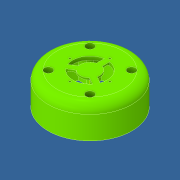
# Autodesk Inventor part: MotorCoverN24_3
Saved by Autodesk Inventor 2016 (Build 200138000, 138)
## iProperties
Created: 2015-09-10
Part Number: MotorCoverN24_3
Material: ABS-Kunststoff
Document SubType Name: Modeling
Designer: 4ndreas
Density: 1.06 g/cm^3
Appearance: Glatt - grün
Mass: 119.697 g
Surface Area: 331.914 cm^2
Volume: 112.922 cm^3
Author: 4ndreas
Autodesk Inventor part; units mm, degrees
ref_plane "YZ Plane" through (0, 0, 0) normal (1, 0, 0) x (0, 1, 0)
ref_plane "XZ Plane" through (0, 0, 0) normal (0, 1, 0) x (-1, 0, 0)
sketch "Skizze1" plane through (0, 0, 0) normal (0, 0, 1) x (1, 0, 0)
  line L0 (24.616, 19.6663) -> (20.7123, 20.7123) projected
  line L1 (20.7123, 20.7123) -> (19.6663, 24.616) projected
  line L2 (19.6663, 24.616) -> (22.524, 27.4737) projected
  line L3 (22.524, 27.4737) -> (26.4277, 26.4277) projected
  line L4 (26.4277, 26.4277) -> (27.4737, 22.524) projected
  line L5 (27.4737, 22.524) -> (24.616, 19.6663) projected
  line L6 (-24.616, -19.6663) -> (-20.7123, -20.7123) projected
  line L7 (-20.7123, -20.7123) -> (-19.6663, -24.616) projected
  line L8 (-19.6663, -24.616) -> (-22.524, -27.4737) projected
  line L9 (-22.524, -27.4737) -> (-26.4277, -26.4277) projected
  line L10 (-26.4277, -26.4277) -> (-27.4737, -22.524) projected
  line L11 (-27.4737, -22.524) -> (-24.616, -19.6663) projected
  line L12 (-20.7123, 20.7123) -> (-24.616, 19.6663) projected
  line L13 (-24.616, 19.6663) -> (-27.4737, 22.524) projected
  line L14 (-27.4737, 22.524) -> (-26.4277, 26.4277) projected
  line L15 (-26.4277, 26.4277) -> (-22.524, 27.4737) projected
  line L16 (-22.524, 27.4737) -> (-19.6663, 24.616) projected
  line L17 (-19.6663, 24.616) -> (-20.7123, 20.7123) projected
  line L18 (19.6663, -24.616) -> (20.7123, -20.7123) projected
  line L19 (20.7123, -20.7123) -> (24.616, -19.6663) projected
  line L20 (24.616, -19.6663) -> (27.4737, -22.524) projected
  line L21 (27.4737, -22.524) -> (26.4277, -26.4277) projected
  line L22 (26.4277, -26.4277) -> (22.524, -27.4737) projected
  line L23 (22.524, -27.4737) -> (19.6663, -24.616) projected
  arc A0 (-23.57, 19.32) -> (-19.32, 23.57) centre (-23.57, 23.57) ccw projected
  line L24 (-19.32, 23.57) -> (-19.32, 32.18) projected
  line L25 (-19.32, 32.18) -> (19.32, 32.18) projected
  line L26 (19.32, 32.18) -> (19.32, 23.57) projected
  arc A1 (19.32, 23.57) -> (23.57, 19.32) centre (23.57, 23.57) ccw projected
  line L27 (23.57, 19.32) -> (32.18, 19.32) projected
  line L28 (32.18, 19.32) -> (32.18, -19.32) projected
  line L29 (32.18, -19.32) -> (23.57, -19.32) projected
  arc A2 (23.57, -19.32) -> (19.32, -23.57) centre (23.57, -23.57) ccw projected
  line L30 (19.32, -23.57) -> (19.32, -32.18) projected
  line L31 (19.32, -32.18) -> (-19.32, -32.18) projected
  line L32 (-19.32, -32.18) -> (-19.32, -23.57) projected
  arc A3 (-19.32, -23.57) -> (-23.57, -19.32) centre (-23.57, -23.57) ccw projected
  line L33 (-23.57, -19.32) -> (-32.18, -19.32) projected
  line L34 (-32.18, -19.32) -> (-32.18, 19.32) projected
  line L35 (-32.18, 19.32) -> (-23.57, 19.32) projected
  circle A4 centre (0, 0) radius 47.5
  circle A5 centre (23.57, -23.57) radius 2
  circle A6 centre (23.57, 23.57) radius 2
  circle A7 centre (-23.57, 23.57) radius 2
  circle A8 centre (-23.57, -23.57) radius 2
  arc A9 (32.18, -19.32) -> (32.18, 19.32) centre (0, 0) ccw
  arc A10 (-19.32, -32.18) -> (19.32, -32.18) centre (0, 0) ccw
  arc A11 (-32.18, 19.32) -> (-32.18, -19.32) centre (0, 0) ccw
  arc A12 (19.32, 32.18) -> (-19.32, 32.18) centre (0, 0) ccw
  point P0 (0, 0)
  dimension "d0" = 4
  dimension "d40" = 95
  constraints: 9 centre point, 8 coincident, 8 point on circle, 3 equal radius
  measures "d0" diameter of A5
  measures "d40" diameter of A4
extrude "Extrusion1" add sketch "Skizze1" along normal blind 32 contours L0 L1 L2 L3 L4 L5 | L6 L7 L8 L9 L10 L11 | L12 L13 L14 L15 L16 L17 | L18 L19 L20 L21 L22 L23 | A4
ref_plane "Arbeitsebene1" through (0, 0, 0) normal (1, 0, 0) x (0, 0, 1)
sketch "Skizze9" plane through (0, 0, 32) normal (0, 0, 1) x (1, 0, 0)
  circle A0 centre (23.57, -23.57) radius 2 projected
  circle A1 centre (-23.57, 23.57) radius 2 projected
  circle A2 centre (-23.57, -23.57) radius 2 projected
  circle A3 centre (23.57, 23.57) radius 2 projected
  circle A4 centre (0, 0) radius 47.5 projected
  line L0 (32.18, -19.32) -> (23.57, -19.32) projected
  arc A5 (23.57, -19.32) -> (19.32, -23.57) centre (23.57, -23.57) ccw projected
  line L1 (19.32, -23.57) -> (19.32, -32.18) projected
  arc A6 (-19.32, -32.18) -> (19.32, -32.18) centre (0, 0) ccw projected
  line L2 (-19.32, -32.18) -> (-19.32, -23.57) projected
  arc A7 (-19.32, -23.57) -> (-23.57, -19.32) centre (-23.57, -23.57) ccw projected
  line L3 (-23.57, -19.32) -> (-32.18, -19.32) projected
  arc A8 (-32.18, 19.32) -> (-32.18, -19.32) centre (0, 0) ccw projected
  line L4 (-32.18, 19.32) -> (-23.57, 19.32) projected
  arc A9 (-23.57, 19.32) -> (-19.32, 23.57) centre (-23.57, 23.57) ccw projected
  line L5 (-19.32, 23.57) -> (-19.32, 32.18) projected
  arc A10 (19.32, 32.18) -> (-19.32, 32.18) centre (0, 0) ccw projected
  line L6 (19.32, 32.18) -> (19.32, 23.57) projected
  arc A11 (19.32, 23.57) -> (23.57, 19.32) centre (23.57, 23.57) ccw projected
  line L7 (23.57, 19.32) -> (32.18, 19.32) projected
  arc A12 (32.18, -19.32) -> (32.18, 19.32) centre (0, 0) ccw projected
  point P0 (0, 0)
extrude "Extrusion6" add sketch "Skizze9" along normal blind 4 contours A4 | L0 A5 L1 A6 L2 A7 L3 A8 L4 A9 L5 A10 L6 A11 L7 A12
fillet "Rundung3" radius 10 1 edges at (-47.5, 0, 36)
sketch "Skizze10" plane through (0, 0, 0) normal (0, 0, -1) x (-1, 0, 0)
  circle A0 centre (-23.57, -23.57) radius 2 projected
  circle A1 centre (23.57, 23.57) radius 2 projected
  circle A2 centre (23.57, -23.57) radius 2 projected
  circle A3 centre (-23.57, 23.57) radius 2 projected
  line L0 (-23.57, -19.32) -> (-32.18, -19.32) projected
  arc A4 (-32.18, 19.32) -> (-32.18, -19.32) centre (0, 0) ccw projected
  line L1 (-32.18, 19.32) -> (-23.57, 19.32) projected
  arc A5 (-23.57, 19.32) -> (-19.32, 23.57) centre (-23.57, 23.57) ccw projected
  line L2 (-19.32, 23.57) -> (-19.32, 32.18) projected
  arc A6 (19.32, 32.18) -> (-19.32, 32.18) centre (0, 0) ccw projected
  line L3 (19.32, 32.18) -> (19.32, 23.57) projected
  arc A7 (19.32, 23.57) -> (23.57, 19.32) centre (23.57, 23.57) ccw projected
  line L4 (23.57, 19.32) -> (32.18, 19.32) projected
  arc A8 (32.18, -19.32) -> (32.18, 19.32) centre (0, 0) ccw projected
  line L5 (32.18, -19.32) -> (23.57, -19.32) projected
  arc A9 (23.57, -19.32) -> (19.32, -23.57) centre (23.57, -23.57) ccw projected
  line L6 (19.32, -23.57) -> (19.32, -32.18) projected
  arc A10 (-19.32, -32.18) -> (19.32, -32.18) centre (0, 0) ccw projected
  line L7 (-19.32, -32.18) -> (-19.32, -23.57) projected
  arc A11 (-19.32, -23.57) -> (-23.57, -19.32) centre (-23.57, -23.57) ccw projected
  circle A12 centre (0, 0) radius 47.5 projected
  point P0 (0, 0)
fillet "Rundung4" radius 5 12 edges at (20.5648, 20.5648, 32) (27.875, 19.32, 32) (19.32, 27.875, 32) (19.32, -27.875, 32) (27.875, -19.32, 32) (20.5648, -20.5648, 32) (-27.875, -19.32, 32) (-19.32, -27.875, 32) (-20.5648, -20.5648, 32) (-19.32, 27.875, 32) (-27.875, 19.32, 32) (-20.5648, 20.5648, 32)
sketch "Skizze11" plane through (0, 0, 36) normal (0, 0, 1) x (1, 0, 0)
  circle A0 centre (23.57, -23.57) radius 2 projected
  circle A1 centre (-23.57, 23.57) radius 2 projected
  circle A2 centre (-23.57, -23.57) radius 2 projected
  circle A3 centre (23.57, 23.57) radius 2 projected
  circle A4 centre (0, 0) radius 37.5 projected
  point P0 (0, 0)
hole "Bohrung2" at (-23.57, 23.57, 36) at (23.57, 23.57, 36) at (23.57, -23.57, 36) at (-23.57, -23.57, 36) direction (0, 0, -1) diameter 4.2 end through all counterbore diameter 9 counterbore depth 6
sketch "Skizze12" plane through (0, 0, 36) normal (0, 0, 1) x (1, 0, 0)
  line L0 (0, -28.2843) -> (28.2843, 0)
  line L1 (28.2843, 0) -> (0, 28.2843)
  line L2 (0, 28.2843) -> (-28.2843, 0)
  line L3 (-28.2843, 0) -> (0, -28.2843)
  line L4 (0, -28.2843) -> (0, 28.2843) construction
  line L5 (28.2843, 0) -> (-28.2843, 0) construction
  arc A0 (25.2121, 27.7597) -> (-25.2121, 27.7597) centre (0, 0) ccw projected
  circle A1 centre (23.57, 23.57) radius 2.1 projected
  circle A2 centre (-23.57, 23.57) radius 2.1 projected
  line L6 (0, -22.6274) -> (22.6274, 0) construction
  line L7 (22.6274, 0) -> (0, 22.6274) construction
  line L8 (0, 22.6274) -> (-22.6274, 0) construction
  line L9 (-22.6274, 0) -> (0, -22.6274) construction
  line L10 (0, -22.6274) -> (0, 22.6274) construction
  line L11 (22.6274, 0) -> (-22.6274, 0) construction
  circle A3 centre (0, 22.6274) radius 1.25
  circle A4 centre (22.6274, 0) radius 1.25
  circle A5 centre (0, -22.6274) radius 1.25
  circle A6 centre (-22.6274, 0) radius 1.25
  circle A7 centre (0, 0) radius 19.5
  circle A8 centre (0, 0) radius 11
  line L12 (-3.1274, 10.5461) -> (3.1274, 10.5461)
  line L13 (3.1274, 10.5461) -> (3.1274, 19.5)
  line L14 (3.1274, 19.5) -> (-3.1274, 19.5)
  line L15 (-3.1274, 19.5) -> (-3.1274, 10.5461)
  line L16 (-3.1274, 10.5461) -> (3.1274, 19.5) construction
  line L17 (3.1274, 10.5461) -> (-3.1274, 19.5) construction
  line L18 (0, 0) -> (-16.8875, -9.75) construction
  line L19 (-15.3238, -12.4584) -> (-7.5694, -7.9814)
  line L20 (-7.5694, -7.9814) -> (-10.6969, -2.5646)
  line L21 (-10.6969, -2.5646) -> (-18.4512, -7.0416)
  line L22 (-18.4512, -7.0416) -> (-15.3238, -12.4584)
  line L23 (-15.3238, -12.4584) -> (-10.6969, -2.5646) construction
  line L24 (-7.5694, -7.9814) -> (-18.4512, -7.0416) construction
  line L25 (0, 0) -> (16.8875, -9.75) construction
  line L26 (15.3238, -12.4584) -> (7.5694, -7.9814)
  line L27 (7.5694, -7.9814) -> (10.6969, -2.5646)
  line L28 (10.6969, -2.5646) -> (18.4512, -7.0416)
  line L29 (18.4512, -7.0416) -> (15.3238, -12.4584)
  line L30 (15.3238, -12.4584) -> (10.6969, -2.5646) construction
  line L31 (7.5694, -7.9814) -> (18.4512, -7.0416) construction
  point P0 (0, 0)
  point P1 (0, 15.023)
  point P2 (-13.0103, -7.5115)
  point P3 (13.0103, -7.5115)
  dimension "d52" = 40
  dimension "d53" = 32
  dimension "d54" = 2.5
  dimension "d55" = 0.5
  dimension "d56" = 22
  dimension "d57" = 120
  dimension "d58" = 120
  constraints: 64 end point, 12 midpoint, 10 parallel, 7 point on circle, 6 centre point, 6 coincident, 5 perpendicular, 4 equal length, 4 point on line, 3 equal radius, 2 collinear, 2 horizontal, 1 tangent, 1 vertical
  measures "d52" distance between parallel lines of L3 L1
  measures "d53" distance between parallel lines of L9 L7
  measures "d54" diameter of A3
  measures "d55" distance edge to line of A7 L1
  measures "d56" diameter of A8
  measures "d57" angle of L18 L4
  measures "d58" angle of L25 L18
extrude "Extrusion7" cut sketch "Skizze12" against normal through all contours A3 | A4 | A5 | A6 | A7 L28 A8 L13 | L13 A8 L15 A7 | A7 L26 A8 L28 | L15 A8 L21 A7 | A7 L19 A8 L26 | L21 A8 L19 A7
extrude "Extrusion8" add sketch "Skizze12" against normal up to surface (4 mm away) contours L13 A8 L15 A7 | A7 L14 L13 | L28 L29 A7 | A7 L26 A8 L28 | A7 L15 L14 | L12 A8 | L29 L26 A7 | L21 A8 L19 A7 | A7 L22 L21 | L19 L22 A7
sketch "Skizze14" plane through (0, 0, 32) normal (0, 0, -1) x (-1, 0, 0)
  arc A0 (18.2326, -6.9154) -> (3.1274, 19.2476) centre (0, 0) ccw projected
  line L0 (18.2326, -6.9154) -> (10.6969, -2.5646) projected
  arc A1 (10.6969, -2.5646) -> (3.1274, 10.5461) centre (0, 0) ccw projected
  line L1 (3.1274, 10.5461) -> (3.1274, 19.2476) projected
  arc A2 (-15.1052, -12.3322) -> (15.1052, -12.3322) centre (0, 0) ccw projected
  line L2 (-15.1052, -12.3322) -> (-7.5694, -7.9814) projected
  arc A3 (-7.5694, -7.9814) -> (7.5694, -7.9814) centre (0, 0) ccw projected
  line L3 (7.5694, -7.9814) -> (15.1052, -12.3322) projected
  circle A4 centre (22.6274, 0) radius 1.25 projected
  circle A5 centre (-22.6274, 0) radius 1.25 projected
  circle A6 centre (0, 22.6274) radius 1.25 projected
  circle A7 centre (0, -22.6274) radius 1.25 projected
  line L4 (14.32, 34.6951) -> (14.32, 23.57) projected
  arc A8 (14.32, 34.6951) -> (-14.32, 34.6951) centre (0, 0) ccw projected
  line L5 (-14.32, 23.57) -> (-14.32, 34.6951) projected
  arc A9 (-23.57, 14.32) -> (-14.32, 23.57) centre (-23.57, 23.57) ccw projected
  line L6 (-34.6951, 14.32) -> (-23.57, 14.32) projected
  arc A10 (-34.6951, 14.32) -> (-34.6951, -14.32) centre (0, 0) ccw projected
  line L7 (-23.57, -14.32) -> (-34.6951, -14.32) projected
  arc A11 (-14.32, -23.57) -> (-23.57, -14.32) centre (-23.57, -23.57) ccw projected
  line L8 (-14.32, -34.6951) -> (-14.32, -23.57) projected
  arc A12 (-14.32, -34.6951) -> (14.32, -34.6951) centre (0, 0) ccw projected
  line L9 (14.32, -23.57) -> (14.32, -34.6951) projected
  arc A13 (23.57, -14.32) -> (14.32, -23.57) centre (23.57, -23.57) ccw projected
  line L10 (34.6951, -14.32) -> (23.57, -14.32) projected
  arc A14 (34.6951, -14.32) -> (34.6951, 14.32) centre (0, 0) ccw projected
  line L11 (23.57, 14.32) -> (34.6951, 14.32) projected
  arc A15 (14.32, 23.57) -> (23.57, 14.32) centre (23.57, 23.57) ccw projected
  line L12 (-3.1274, 19.2476) -> (-3.1274, 10.5461) projected
  arc A16 (-3.1274, 10.5461) -> (-10.6969, -2.5646) centre (0, 0) ccw projected
  line L13 (-10.6969, -2.5646) -> (-18.2326, -6.9154) projected
  arc A17 (-3.1274, 19.2476) -> (-18.2326, -6.9154) centre (0, 0) ccw projected
  circle A18 centre (0, 0) radius 19.5
  point P0 (0, 0)
  constraints: 1 centre point, 1 coincident, 1 concentric
extrude "Extrusion9" cut sketch "Skizze14" against normal blind 2 contours A18 L3 A3 L2 L13 A16 L12 L1 A1 L0
chamfer "Fase1" distance 2 angle 45 3 edges at (0, 19.5, 34) (-16.8875, -9.75, 34) (16.8875, -9.75, 34)
equation "\"d58\" = d57"
